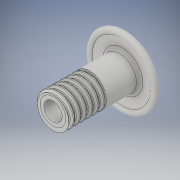
# Autodesk Inventor part: Kabelzugentlastung
Saved by Autodesk Inventor 2018.2 (Build 222227000, 227)
## iProperties
Created: 2018-01-25
Part Number: Kabelzugentlastung
Material: Generisch
Document SubType Name: Modeling
Designer: JochenAlt
Density: 1 g/cm^3
Appearance: Vorgabe
Author: JochenAlt
Autodesk Inventor part; units mm, degrees
ref_plane "YZ Plane" through (0, 0, 0) normal (1, 0, 0) x (0, 1, 0)
ref_plane "XZ Plane" through (0, 0, 0) normal (0, 1, 0) x (-1, 0, 0)
ref_plane "XY Plane" through (0, 0, 0) normal (0, 0, 1) x (1, 0, 0)
sketch "Skizze1" plane through (0, 0, 0) normal (0, 0, 1) x (1, 0, 0)
  line L0 (0, 77.3285) -> (0, -12.8881) construction
  line L1 (-5.6319, 0) -> (21.6987, 0) construction
  arc A0 (10.3306, 60.1189) -> (10.3306, 60.1189) centre (0, 0) ccw
  arc A1 (10.6694, 62.09) -> (3.528, 62.9011) centre (0, 0) ccw
  arc A2 (10.3306, 60.1189) -> (10.6694, 62.09) centre (10.5, 61.1044) ccw
  line L2 (5.5, 62.9404) -> (5.5, 63.1904)
  line L3 (4.25, 64.4404) -> (4.25, 64.4404)
  line L4 (5.5, 60.0492) -> (5.5, 49.7515)
  line L5 (3, 62.4019) -> (3, 38.0492)
  line L6 (5.5, 49.7515) -> (5.5, 49.7515)
  line L7 (5.5, 49.7515) -> (5.5, 38.0492)
  line L8 (5.5, 38.0492) -> (3, 38.0492)
  arc A3 (9.6129, 60.6428) -> (6.6076, 61.0434) centre (0, 0) ccw
  arc A4 (6.6076, 61.0434) -> (5.5, 60.0492) centre (6.5, 60.0492) ccw
  arc A5 (9.6129, 60.6428) -> (10.3306, 60.1189) centre (10.5, 61.1044) ccw
  arc A6 (3.528, 62.9011) -> (3, 62.4019) centre (3.5, 62.4019) ccw
  point P0 (-1.7275, 62.9763)
  point P1 (17.7943, 58.3469)
  point P2 (4.8231, 61.4229)
  point P3 (4.8231, 61.4229)
  point P4 (3, 62.9285)
  point P5 (9.5, 60.6606)
  point P6 (10, 60.1747)
  dimension "d3" = 2
  dimension "d4" = 61
  dimension "d6" = 5.5
  dimension "d60" = 5
  dimension "d370" = 2.5
  dimension "d373" = 2.5
  dimension "d547" = 61.4
  dimension "d551" = 9.5
  dimension "d552" = 1
  dimension "d553" = 22
  dimension "d573" = 0.5
  constraints: 19 point on circle, 14 end point, 7 centre point, 7 tangent, 4 coincident, 3 horizontal, 2 vertical, 1 collinear, 1 equal radius, 1 perpendicular, 1 point on line, 5 other
  measures "d3" radial gap between concentric circles of A1 A0
  measures "d4" radius of A0
  measures "d6" distance between parallel lines of L2 L0
  measures "d60" horizontal distance of A2.centre L2.start
  measures "d370" distance between parallel lines of L7 L5
  measures "d373" distance between parallel lines of L5 L4
  measures "d547" radius of A3
  measures "d551" distance from line of point (9.5, 60.661) L0
  measures "d552" radius of A4
  measures "d553" distance from line of L8 A4.centre
  measures "d573" radius of A6
revolve "Umdrehung1" add sketch "Skizze1" angle 360 about axis through (0, 0, 0) along (0, -1, 0) picked at (3.8333, 49.5756) contours A5 A3 A4 A0 L5 A6 A1 A2 | A0 A4 L4 L7 L8 L5
thread "Gewinde5" size "M16x2" class "6g" standard "ANSI Metric M Profile" length 12
sketch "Skizze87" plane through (0, 38.1498, 0) normal (-1, 0, 0) x (0, 0, 1)
  line L0 (5.5, 0) -> (5.5, 12)
  line L1 (5.5, 12) -> (4.1948, 12)
  line L2 (4.1948, 12) -> (4.1948, 0)
  line L3 (4.1948, 0) -> (5.5, 0)
  line L4 (0, -2.4) -> (0, 14.4) projected
  constraints: 8 end point
revolve "Umdrehung56" cut sketch "Skizze87" angle 360 about axis through (0, 38.1498, 0) along (0, 1, 0)
sketch "Skizze88" plane through (0, 38.1498, 0) normal (-1, 0, 0) x (0, 0, 1)
  line L0 (5.5, 0) -> (5.5, 12)
  line L1 (5.5, 12) -> (4.1948, 12)
  line L2 (4.1948, 12) -> (4.1948, 0)
  line L3 (4.1948, 0) -> (5.5, 0)
  line L4 (0, -2.4) -> (0, 14.4) projected
  constraints: 8 end point
revolve "Umdrehung57" add sketch "Skizze88" angle 360 about axis through (0, 38.1498, 0) along (0, 1, 0) separate body
sketch "Skizze86" plane through (0, 38.1498, 0) normal (1, 0, 0) x (0, 1, 0)
  line L0 (-1.2688, -4.8235) -> (-1.0001, -4.8235) construction
  line L1 (0.2685, -5.3749) -> (-0.0001, -5.6951) construction
  line L2 (-2.0001, -5.6951) -> (-2.2688, -5.3749) construction
  line L3 (-0.7315, -4.8235) -> (-1.0001, -4.5033) construction
  line L4 (-1.0001, -4.5033) -> (-1.2688, -4.8235) construction
  line L5 (-2.0001, -5.6951) -> (-1.7315, -5.3749) construction
  line L6 (-0.7315, -4.8235) -> (-0.2688, -5.3749)
  line L7 (-2.2688, -5.3749) -> (-1.7315, -5.3749) construction
  arc A0 (-2.2688, -5.3749) -> (-2.0001, -5.5002) centre (-2.0001, -5.1495) ccw construction
  line L8 (0.2685, -5.3749) -> (-0.2688, -5.3749) construction
  line L9 (-2.0001, -5.6951) -> (-2.0001, -5.3749) construction
  line L10 (-0.0001, -5.6951) -> (-0.0001, -5.3749) construction
  line L11 (-1.0001, -4.5033) -> (-1.0001, -4.6982) construction
  line L12 (-2.0001, -5.5002) -> (-0.0001, -5.5002)
  arc A1 (-2.0001, -5.5002) -> (-1.7315, -5.3749) centre (-2.0001, -5.1495) ccw
  line L13 (-0.2688, -5.3749) -> (-0.0001, -5.6951) construction
  line L14 (-1.7315, -5.3749) -> (-1.2688, -4.8235)
  line L15 (-0.0001, -0.0002) -> (-0.0001, 0.0177)
  line L16 (-0.0001, 0.0177) -> (-0.0001, -0.0002)
  line L17 (-0.0001, -0.0002) -> (0.0334, -0.0002)
  arc A2 (-0.2688, -5.3749) -> (-0.0001, -5.5002) centre (-0.0001, -5.1495) ccw
  arc A3 (-0.0001, -5.5002) -> (0.2685, -5.3749) centre (-0.0001, -5.1495) ccw construction
  arc A4 (-1.0001, -4.6982) -> (-1.2688, -4.8235) centre (-1.0001, -5.0489) ccw
  arc A5 (-0.7315, -4.8235) -> (-1.0001, -4.6982) centre (-1.0001, -5.0489) ccw
  line L18 (-1.0001, -4.6982) -> (-1.0001, -4.8235) construction
  line L19 (-1.0001, -4.8235) -> (-0.7315, -4.8235) construction
  dimension "d554" = 80
  dimension "d555" = 0.3202
  dimension "d556" = 0.3202
  dimension "Skizze86_ThreadOffset" = 0
  dimension "Skizze86_MajorRadius" = 5.5
  dimension "d559" = 2
  dimension "Skizze86_MinorRadius" = 4.698
  constraints: 40 end point, 12 point on circle, 10 parallel, 8 tangent, 6 centre point, 6 collinear, 2 midpoint, 2 point on line, 1 horizontal, 1 perpendicular, 3 other
  measures "d554" angle of L6 L14
  measures "d555" distance of L3.end L0.end
  measures "d556" distance of L1.end L10.end
  measures "Skizze86_ThreadOffset" distance between parallel lines of L15 L10
  measures "Skizze86_MajorRadius" distance from line of L12 L15.start
  measures "d559" distance from line of L1.end L9
  measures "Skizze86_MinorRadius" distance edge to line of A5 L17
coil "Spirale28" sketch "Skizze86" operation cut axis through (0, 38.1498, 0) along (0, 1, 0) pitch 2.002 turns 7.992008 hand right bodies 2
sketch "Skizze91" plane through (0, 38.0492, 0) normal (0, -1, 0) x (1, 0, 0)
  circle A0 centre (0, 0) radius 5.5
  constraints: 1 centre point, 1 coincident
extrude "Extrusion2" cut sketch "Skizze91" against normal up to surface (0.1006 mm away) bodies 1
equation "\"d370\" = d373"
equation "\"d26\" = 60deg"
equation "\"Skizze2_Pitch\" = 1"
equation "\"d47\" = 60deg"
equation "\"Skizze5_Pitch\" = 2"
equation "\"d70\" = 60deg"
equation "\"Skizze8_Pitch\" = 2"
equation "\"d90\" = 60deg"
equation "\"Skizze11_Pitch\" = 2"
equation "\"d111\" = 60deg"
equation "\"Skizze14_Pitch\" = 2.54"
equation "\"d130\" = 60deg"
equation "\"Skizze17_Pitch\" = 2"
equation "\"d149\" = 60deg"
equation "\"Skizze20_Pitch\" = 1.33684"
equation "\"d168\" = 60deg"
equation "\"Skizze23_Pitch\" = 1.3"
equation "\"d187\" = 60deg"
equation "\"Skizze26_Pitch\" = 1.33684"
equation "\"d206\" = 60deg"
equation "\"Skizze29_Pitch\" = 1.33684"
equation "\"d225\" = 60deg"
equation "\"Skizze32_Pitch\" = 2.6"
equation "\"d244\" = 60deg"
equation "\"Skizze35_Pitch\" = 1.5"
equation "\"d263\" = 60deg"
equation "\"Skizze38_Pitch\" = 2.54"
equation "\"d282\" = 60deg"
equation "\"Skizze42_Pitch\" = 2.30909"
equation "\"d301\" = 60deg"
equation "\"Skizze46_Pitch\" = 3"
equation "\"d320\" = 60deg"
equation "\"Skizze49_Pitch\" = 2"
equation "\"d339\" = 60deg"
equation "\"Skizze53_Pitch\" = 1"
equation "\"d358\" = 60deg"
equation "\"Skizze56_Pitch\" = 2"
equation "\"d383\" = 60deg"
equation "\"Skizze59_Pitch\" = 1.5"
equation "\"d402\" = 60deg"
equation "\"Skizze62_Pitch\" = 1.5"
equation "\"d421\" = 60deg"
equation "\"Skizze65_Pitch\" = 5"
equation "\"d440\" = 60deg"
equation "\"Skizze68_Pitch\" = 5"
equation "\"d459\" = 60deg"
equation "\"Skizze71_Pitch\" = 3.6"
equation "\"d478\" = 60deg"
equation "\"Skizze74_Pitch\" = 2.2"
equation "\"d497\" = 60deg"
equation "\"Skizze77_Pitch\" = 2.2"
equation "\"d516\" = 60deg"
equation "\"Skizze80_Pitch\" = 2"
equation "\"d535\" = 60deg"
equation "\"Skizze83_Pitch\" = 2"
equation "\"d561\" = 60deg"
equation "\"Skizze86_Pitch\" = 2"
